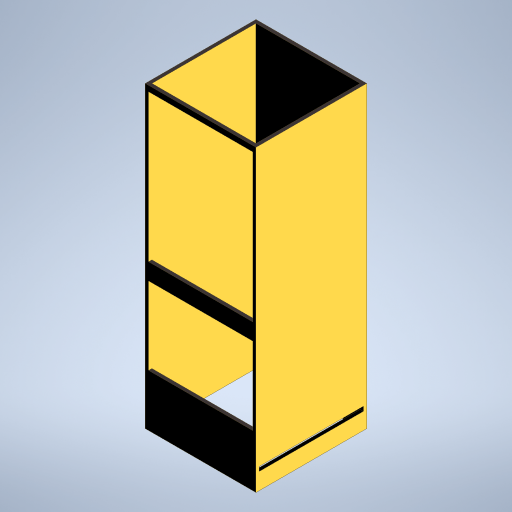
# Autodesk Inventor part: FLU-ShaftRS3
Saved by Autodesk Inventor 2024.3 (Build 283343000, 343)
## iProperties
Created: 2025-06-13
Part Number: FLU-ShaftRS3
Material: Silver
Document SubType Name: Modeling
Designer: ajclo
Density: 10.49 g/cm^3
Appearance: Silver
Author: ajclo
Autodesk Inventor part; units mm, degrees
ref_plane "YZ Plane" through (0, 0, 0) normal (1, 0, 0) x (0, 1, 0)
ref_plane "XZ Plane" through (0, 0, 0) normal (0, 1, 0) x (-1, 0, 0)
ref_plane "XY Plane" through (0, 0, 0) normal (0, 0, 1) x (1, 0, 0)
sketch "Sketch1" plane through (0, 0, 0) normal (0, 1, 0) x (-1, 0, 0)
  line L0 (50, 50) -> (-50, 50)
  line L1 (-50, 50) -> (-50, -50)
  line L2 (-50, -50) -> (50, -50)
  line L3 (50, -50) -> (50, 50)
  line L4 (50, 50) -> (-50, -50) construction
  line L5 (-50, 50) -> (50, -50) construction
  line L6 (-47, 47) -> (47, 47)
  line L7 (47, 47) -> (47, -47)
  line L8 (47, -47) -> (-47, -47)
  line L9 (-47, -47) -> (-47, 47)
  line L10 (-47, 47) -> (47, -47) construction
  line L11 (47, 47) -> (-47, -47) construction
  point P0 (0, 0)
  dimension "d0" = 100
  dimension "d1" = 100
  dimension "d2" = 3
  dimension "d3" = 3
  constraints: 24 end point, 4 midpoint, 4 parallel, 2 horizontal, 2 perpendicular, 1 point on line
  measures "d0" distance of L2.end L0.start
  measures "d1" distance of L1.end L2.end
  measures "d2" distance between parallel lines of L2 L8
  measures "d3" distance between parallel lines of L7 L3
extrude "Extrusion1" add sketch "Sketch1" along normal blind 270
sketch "Sketch2" plane through (-50, 0, 50) normal (0, 0, 1) x (1, 0, 0)
  line L0 (3, 265) -> (97, 265)
  line L1 (97, 265) -> (97, 132)
  line L2 (97, 132) -> (3, 132)
  line L3 (3, 132) -> (3, 265)
  line L4 (0, 0) -> (0, 270) projected
  line L5 (0, 270) -> (100, 270) projected
  line L6 (3, 117) -> (97, 117)
  line L7 (97, 117) -> (97, 47)
  line L8 (97, 47) -> (3, 47)
  line L9 (3, 47) -> (3, 117)
  line L10 (100, 0) -> (100, 270) projected
  point P0 (50, 0)
  point P1 (50, 270)
  point P2 (50, 265)
  dimension "d6" = 94
  dimension "d7" = 3
  dimension "d8" = 5
  dimension "d9" = 133
  dimension "d10" = 70
  dimension "d11" = 15
  dimension "d12" = 3
  constraints: 16 end point, 4 parallel, 2 horizontal, 2 midpoint, 2 perpendicular, 1 collinear
  measures "d6" distance of L0.start L0.end
  measures "d7" distance between parallel lines of L4 L3
  measures "d8" distance from line of point (50, 270) L0
  measures "d9" distance from line of point (50, 265) L2
  measures "d10" distance of L6.end L7.end
  measures "d11" distance between parallel lines of L6 L2
  measures "d12" distance between parallel lines of L10 L7
extrude "Extrusion2" cut sketch "Sketch2" against normal blind 10
sketch "Sketch10" plane through (50, 0, 50) normal (1, 0, 0) x (0, 0, -1)
  line L0 (3, 0) -> (3, 47) projected
  line L1 (97, 0) -> (97, 270) projected
  line L2 (3, 19) -> (97, 19)
  line L3 (97, 19) -> (97, 15)
  line L4 (97, 15) -> (3, 15)
  line L5 (3, 15) -> (3, 19)
  line L6 (0, 0) -> (100, 0) projected
  point P0 (50, 0)
  point P1 (3, 15)
  dimension "d46" = 4
  dimension "d49" = 15
  constraints: 8 end point, 2 parallel, 2 point on line, 1 horizontal, 1 perpendicular
  measures "d46" distance between parallel lines of L4 L2
  measures "d49" distance between parallel lines of L6 L4
extrude "Extrusion10" cut sketch "Sketch10" against normal blind 10 contours L0 L2 L1 L4
equation "\"d1\" = d0"
equation "\"d12\" = d7"
body "Solid1"
